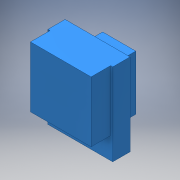
# Autodesk Inventor part: Modulo
Saved by Autodesk Inventor 2016 (Build 200138000, 138)
## iProperties
Created: 2017-05-09
Part Number: Modulo
Material: Generic
Document SubType Name: Modeling
Designer: rdiaz
Density: 1 g/cm^3
Appearance: Cyan
Author: rdiaz
Autodesk Inventor part; units mm, degrees
ref_plane "YZ Plane" through (0, 0, 0) normal (1, 0, 0) x (0, 1, 0)
ref_plane "XZ Plane" through (0, 0, 0) normal (0, 1, 0) x (-1, 0, 0)
ref_plane "XY Plane" through (0, 0, 0) normal (0, 0, 1) x (1, 0, 0)
sketch "Sketch1" plane through (0, 0, 0) normal (0, 1, 0) x (-1, 0, 0)
  line L0 (12.65, 7.65) -> (-12.65, 7.65)
  line L1 (-12.65, 7.65) -> (-12.65, -7.65)
  line L2 (-12.65, -7.65) -> (12.65, -7.65)
  line L3 (12.65, -7.65) -> (12.65, 7.65)
  point P0 (0, 0)
  point P1 (0, 7.65)
  point P2 (12.65, 0)
  dimension "d0" = 15.3
  dimension "d1" = 25.3
  constraints: 8 end point, 2 midpoint, 2 parallel, 1 horizontal, 1 horizontal alignment, 1 perpendicular, 1 vertical alignment
  measures "d0" distance of L2.end L0.start
  measures "d1" distance of L1.end L2.end
extrude "Extrusion1" add sketch "Sketch1" along normal blind 10
sketch "Sketch2" plane through (0, 10, 0) normal (0, 1, 0) x (1, 0, 0)
  line L0 (-12.65, -7.65) -> (12.65, -7.65) projected
  line L1 (12.65, -7.65) -> (12.65, 7.65) projected
  line L2 (12.65, 7.65) -> (-12.65, 7.65) projected
  line L3 (-12.65, 7.65) -> (-12.65, -7.65) projected
  line L4 (19, 15) -> (-19, 15)
  line L5 (-19, 15) -> (-19, -15)
  line L6 (-19, -15) -> (19, -15)
  line L7 (19, -15) -> (19, 15)
  point P0 (0, 0)
  point P1 (19, 0)
  point P2 (0, 15)
  dimension "d4" = 30
  dimension "d5" = 38
  constraints: 8 end point, 2 midpoint, 2 parallel, 1 horizontal, 1 horizontal alignment, 1 perpendicular, 1 vertical alignment
  measures "d4" distance of L6.end L4.start
  measures "d5" distance of L5.end L6.end
extrude "Extrusion2" add sketch "Sketch2" along normal blind 8 contours L3 L2 L1 L0 | L7 L6 L5 L4
sketch "Sketch3" plane through (0, 18, 0) normal (0, 1, 0) x (1, 0, 0)
  line L0 (19, 15) -> (-19, 15) projected
  line L1 (-19, 15) -> (-19, -15) projected
  line L2 (-19, -15) -> (19, -15) projected
  line L3 (19, -15) -> (19, 15) projected
  line L4 (-19, -14) -> (9, -14)
  line L5 (9, -14) -> (9, 14)
  line L6 (9, 14) -> (-19, 14)
  line L7 (-19, 14) -> (-19, -14)
  line L8 (-19, -14) -> (-19, 0) construction
  line L9 (-19, 0) -> (9, 0) construction
  point P0 (0, 0)
  point P1 (-19, 0)
  point P2 (-5, 0)
  dimension "d8" = 28
  dimension "d9" = 28
  dimension "d10" = 14
  constraints: 12 end point, 4 midpoint, 2 horizontal alignment, 2 parallel, 1 collinear, 1 horizontal, 1 perpendicular
  measures "d8" distance of L5.end L6.end
  measures "d9" distance of L6.end L4.start
  measures "d10" distance of L4.start L8.end
extrude "Extrusion3" add sketch "Sketch3" along normal blind 9 contours L6 L5 L4 L1
body "Solid1"
